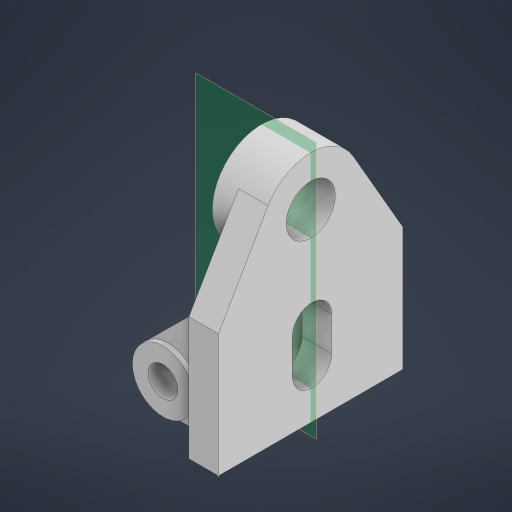
# Autodesk Inventor part: Część23
Saved by Autodesk Inventor 2023 (Build 270158000, 158)
## iProperties
Created: 2023-05-09
Part Number: Część23
Material: Ogólny
Document SubType Name: Modeling
Designer: Adam
Density: 1 g/cm^3
Appearance: Domyślna
Author: Adam
Autodesk Inventor part; units mm, degrees
ref_plane "YZ Plane" through (0, 0, 0) normal (1, 0, 0) x (0, 1, 0)
ref_plane "XZ Plane" through (0, 0, 0) normal (0, 1, 0) x (-1, 0, 0)
ref_plane "XY Plane" through (0, 0, 0) normal (0, 0, 1) x (1, 0, 0)
sketch "Szkic1" plane through (0, 0, 0) normal (1, 0, 0) x (0, 1, 0)
  line L0 (0, 0) -> (50, 0)
  line L1 (50, 0) -> (50, -75)
  line L2 (50, -75) -> (0, -75)
  line L3 (0, -75) -> (0, 0)
  circle A0 centre (75, -37.5) radius 20
  line L4 (50, 0) -> (84.9897, -20.1735)
  line L5 (50, -75) -> (84.9897, -54.8265)
  dimension "d0" = 50
  dimension "d1" = 75
  dimension "d2" = 40
  dimension "d3" = 25
  dimension "d4" = 37.5
  constraints: 12 end point, 2 parallel, 2 point on circle, 2 tangent, 1 centre point, 1 horizontal, 1 perpendicular
  measures "d0" distance of L1.end L2.end
  measures "d1" distance of L0.end L1.end
  measures "d2" diameter of A0
  measures "d3" distance from line of L1 A0.centre
  measures "d4" distance from line of L0 A0.centre
extrude "Wyciągnięcie proste1" add sketch "Szkic1" along normal blind 12
sketch "Szkic2" plane through (12, 0, 0) normal (1, 0, 0) x (0, 0, -1)
  point P0 (0, 0)
sketch "Szkic3" plane through (0, 0, 0) normal (-1, 0, 0) x (0, 0, 1)
  arc A0 (-20.1735, 84.9897) -> (-54.8265, 84.9897) centre (-37.5, 75) ccw projected
  circle A1 centre (-37.5, 75) radius 20
  point P0 (0, 0)
  point P1 (-54.8265, 84.9897)
  point P2 (-20.1735, 84.9897)
  dimension "d7" = 40
  constraints: 1 centre point, 1 coincident
  measures "d7" diameter of A1
extrude "Wyciągnięcie proste2" add sketch "Szkic3" along normal blind 8
sketch "Szkic4" plane through (0, 0, 0) normal (-1, 0, 0) x (0, 0, 1)
  circle A0 centre (-38, 34) radius 8
  circle A1 centre (-38, 20) radius 8
  line L0 (-46, 34) -> (-46, 20)
  line L1 (-30, 34) -> (-30, 20)
  line L2 (0, 0) -> (-75, 0) projected
  dimension "d10" = 16
  dimension "d11" = 16
  dimension "d12" = 14
  dimension "d13" = 20
  constraints: 4 end point, 4 point on circle, 2 centre point, 2 tangent, 1 parallel
  measures "d10" diameter of A0
  measures "d11" diameter of A1
  measures "d12" distance of A1.centre A0.centre
  measures "d13" distance from line of A1.centre L2
extrude "Wyciągnięcie proste3" cut sketch "Szkic4" against normal through all
sketch "Szkic5" plane through (-8, 75, -37.5) normal (-1, 0, 0) x (0, 0, 1)
  point P0 (37.5, -75)
  point P1 (0, 0)
hole "Otwór1" at (-8, 75, -37.5) direction (1, 0, 0) diameter 20 end through all
ref_plane "Płaszczyzna konstrukcyjna1" through (0, 0, -63.5) normal (0, 0, -1) x (-1, 0, 0)
sketch "Szkic6" plane through (0, 0, -63.5) normal (0, 0, -1) x (-1, 0, 0)
  circle A0 centre (20, 12.5) radius 12.5
  line L0 (0, 50) -> (-12, 50) projected
  line L1 (0, 50) -> (28.8115, 21.3661)
  line L2 (0, 0) -> (0, 50) projected
  line L3 (0, 0) -> (20, 0)
  dimension "d24" = 25
  dimension "d25" = 20
  constraints: 4 end point, 2 point on circle, 2 tangent, 1 centre point, 1 horizontal
  measures "d24" diameter of A0
  measures "d25" distance from line of L2 A0.centre
extrude "Wyciągnięcie proste4" add sketch "Szkic6" against normal blind 10
ref_plane "Płaszczyzna konstrukcyjna2" through (0, 0, -37.5) normal (0, 0, -1) x (-1, 0, 0)
sketch "Szkic7" plane through (0, 0, -63.5) normal (0, 0, -1) x (-1, 0, 0)
  arc A0 (20, 0) -> (28.8115, 21.3661) centre (20, 12.5) ccw projected
  circle A1 centre (20, 12.5) radius 12.5
  point P0 (0, 0)
  dimension "d28" = 25
  constraints: 1 centre point, 1 coincident
  measures "d28" diameter of A1
extrude "Wyciągnięcie proste5" add sketch "Szkic7" along normal blind 2
sketch "Szkic8" plane through (-20, 12.5, -65.5) normal (0, 0, -1) x (-1, 0, 0)
  point P0 (-20, -12.5)
  point P1 (0, 0)
hole "Otwór2" at (-20, 12.5, -65.5) direction (0, 0, 1) diameter 12 end through all
mirror "Odbij1" about plane through (0, 0, -37.5) normal (0, 0, -1) of "Wyciągnięcie proste4", "Wyciągnięcie proste5", "Otwór2"
fillet "Zaokrąglenie1" radius 1 4 edges at (0, 25, -63.5) (0, 25, -21.5) (0, 25, -11.5) (0, 25, -53.5)
